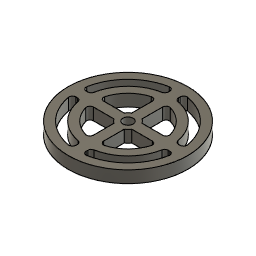
ruote_1.0 v1 (Autodesk Fusion 360 design; units mm, degrees)
Autodesk Fusion 360 part; units mm, degrees
sketch "Sketch1" plane through (0, 0, 0) normal (0, 1, 0) x (1, 0, 0)
  arc A0 (3, -5.1962) -> (5.1962, -3) centre (0, 0) ccw
  arc A1 (5.1962, 3) -> (3, 5.1962) centre (0, 0) ccw
  arc A2 (-3, 5.1962) -> (-5.1962, 3) centre (0, 0) ccw
  arc A3 (-5.1962, -3) -> (-3, -5.1962) centre (0, 0) ccw
  line L0 (-3, -5.1962) -> (-3, -17.2916)
  line L1 (3, -5.1962) -> (3, -17.2916)
  arc A4 (5.5556, -19.2129) -> (19.2129, -5.5556) centre (0, 0) ccw
  line L2 (-5.1962, 3) -> (-17.2916, 3)
  line L3 (-5.1962, -3) -> (-17.2916, -3)
  arc A5 (-19.2129, -5.5556) -> (-5.5556, -19.2129) centre (0, 0) ccw
  arc A6 (19.2129, 5.5556) -> (5.5556, 19.2129) centre (0, 0) ccw
  arc A7 (-5.5556, 19.2129) -> (-19.2129, 5.5556) centre (0, 0) ccw
  line L4 (-3, 5.1962) -> (-3, 17.2916)
  line L5 (3, 5.1962) -> (3, 17.2916)
  line L6 (5.1962, 3) -> (17.2916, 3)
  line L7 (5.1962, -3) -> (17.2916, -3)
  line L8 (-3, -26.533) -> (-3, -27.55)
  line L9 (3, -26.533) -> (3, -27.55)
  line L10 (-26.533, 3) -> (-27.55, 3)
  line L11 (-26.533, -3) -> (-27.55, -3)
  arc A8 (-29.5178, -5.3571) -> (-5.3571, -29.5178) centre (0, 0) ccw
  arc A9 (-24.5676, -4.6296) -> (-4.6296, -24.5676) centre (0, 0) ccw
  arc A10 (4.6296, -24.5676) -> (24.5676, -4.6296) centre (0, 0) ccw
  arc A11 (5.3571, -29.5178) -> (29.5178, -5.3571) centre (0, 0) ccw
  line L12 (26.533, -3) -> (27.55, -3)
  line L13 (26.533, 3) -> (27.55, 3)
  line L14 (-3, 26.533) -> (-3, 27.55)
  line L15 (3, 26.533) -> (3, 27.55)
  arc A12 (29.5178, 5.3571) -> (5.3571, 29.5178) centre (0, 0) ccw
  arc A13 (-5.3571, 29.5178) -> (-29.5178, 5.3571) centre (0, 0) ccw
  arc A14 (24.5676, 4.6296) -> (4.6296, 24.5676) centre (0, 0) ccw
  arc A15 (-4.6296, 24.5676) -> (-24.5676, 4.6296) centre (0, 0) ccw
  circle A16 centre (0, 0) radius 35
  circle A17 centre (0, 0) radius 3
  arc A18 (-5.3571, -29.5178) -> (-3, -27.55) centre (-5, -27.55) ccw
  arc A19 (-3, -26.533) -> (-4.6296, -24.5676) centre (-5, -26.533) ccw
  arc A20 (-24.5676, -4.6296) -> (-26.533, -3) centre (-26.533, -5) ccw
  arc A21 (-27.55, -3) -> (-29.5178, -5.3571) centre (-27.55, -5) ccw
  arc A22 (-29.5178, 5.3571) -> (-27.55, 3) centre (-27.55, 5) ccw
  arc A23 (-26.533, 3) -> (-24.5676, 4.6296) centre (-26.533, 5) ccw
  arc A24 (-4.6296, 24.5676) -> (-3, 26.533) centre (-5, 26.533) ccw
  arc A25 (-3, 27.55) -> (-5.3571, 29.5178) centre (-5, 27.55) ccw
  arc A26 (5.3571, 29.5178) -> (3, 27.55) centre (5, 27.55) ccw
  arc A27 (3, 26.533) -> (4.6296, 24.5676) centre (5, 26.533) ccw
  arc A28 (24.5676, 4.6296) -> (26.533, 3) centre (26.533, 5) ccw
  arc A29 (27.55, 3) -> (29.5178, 5.3571) centre (27.55, 5) ccw
  arc A30 (29.5178, -5.3571) -> (27.55, -3) centre (27.55, -5) ccw
  arc A31 (26.533, -3) -> (24.5676, -4.6296) centre (26.533, -5) ccw
  arc A32 (4.6296, -24.5676) -> (3, -26.533) centre (5, -26.533) ccw
  arc A33 (3, -27.55) -> (5.3571, -29.5178) centre (5, -27.55) ccw
  arc A34 (3, -17.2916) -> (5.5556, -19.2129) centre (5, -17.2916) ccw
  arc A35 (-5.5556, -19.2129) -> (-3, -17.2916) centre (-5, -17.2916) ccw
  arc A36 (-17.2916, -3) -> (-19.2129, -5.5556) centre (-17.2916, -5) ccw
  arc A37 (-19.2129, 5.5556) -> (-17.2916, 3) centre (-17.2916, 5) ccw
  arc A38 (-3, 17.2916) -> (-5.5556, 19.2129) centre (-5, 17.2916) ccw
  arc A39 (5.5556, 19.2129) -> (3, 17.2916) centre (5, 17.2916) ccw
  arc A40 (17.2916, 3) -> (19.2129, 5.5556) centre (17.2916, 5) ccw
  arc A41 (19.2129, -5.5556) -> (17.2916, -3) centre (17.2916, -5) ccw
  dimension "d2" = 2
  constraint vertical L1
  constraint vertical L0
  constraint horizontal L7
  constraint horizontal L6
  constraint perpendicular L5 L6
  constraint parallel L4 L5
  constraint horizontal L2
  constraint parallel L2 L3
  constraint coincident A3.start A0
  constraint concentric A0 A1
  constraint concentric A1 A2
  constraint concentric A2 A3
  constraint concentric A4 A6
  constraint concentric A5 A6
  constraint concentric A6 A7
  constraint concentric A4 A8
  constraint concentric A3 A9
  constraint vertical L8
  constraint parallel L8 L9
  constraint parallel L7 L12
  constraint perpendicular L5 L13
  constraint parallel L5 L15
  constraint vertical L14
  constraint parallel L2 L10
  constraint parallel L3 L11
  constraint concentric A8 A11
  constraint concentric A9 A10
  constraint concentric A10 A14
  constraint concentric A11 A12
  constraint concentric A12 A13
  constraint concentric A14 A15
  constraint concentric A14 A16
  constraint concentric A8 A17
  constraint tangent L8 A18
  constraint tangent A8 A18
  constraint tangent A9 A19
  constraint tangent L8 A19
  constraint equal A18 A19
  constraint tangent L11 A20
  constraint tangent A9 A20
  constraint equal A18 A20
  constraint tangent L11 A21
  constraint tangent A8 A21
  constraint equal A18 A21
  constraint tangent L10 A22
  constraint tangent A13 A22
  constraint equal A18 A22
  constraint tangent L10 A23
  constraint tangent A15 A23
  constraint equal A18 A23
  constraint tangent A15 A24
  constraint tangent L14 A24
  constraint equal A18 A24
  constraint tangent L14 A25
  constraint tangent A13 A25
  constraint equal A18 A25
  constraint tangent L15 A26
  constraint tangent A12 A26
  constraint equal A18 A26
  constraint tangent A14 A27
  constraint tangent L15 A27
  constraint equal A18 A27
  constraint tangent L13 A28
  constraint tangent A14 A28
  constraint equal A18 A28
  constraint tangent L13 A29
  constraint tangent A12 A29
  constraint equal A18 A29
  constraint tangent A11 A30
  constraint tangent L12 A30
  constraint equal A18 A30
  constraint tangent A10 A31
  constraint tangent L12 A31
  constraint equal A18 A31
  constraint tangent L9 A32
  constraint tangent A10 A32
  constraint equal A18 A32
  constraint tangent L9 A33
  constraint tangent A11 A33
  constraint equal A18 A33
  constraint tangent L1 A34
  constraint tangent A4 A34
  constraint equal A18 A34
  constraint tangent L0 A35
  constraint tangent A5 A35
  constraint equal A18 A35
  constraint tangent L3 A36
  constraint tangent A5 A36
  constraint equal A18 A36
  constraint tangent L2 A37
  constraint tangent A7 A37
  constraint equal A18 A37
  constraint tangent A7 A38
  constraint tangent L4 A38
  constraint equal A18 A38
  constraint tangent A6 A39
  constraint tangent L5 A39
  constraint equal A18 A39
  constraint tangent A6 A40
  constraint tangent L6 A40
  constraint equal A18 A40
  constraint tangent A4 A41
  constraint tangent L7 A41
  constraint equal A18 A41
  measures "d2" radius of A18
extrude "Extrude1" add sketch "Sketch1" along normal blind 7
